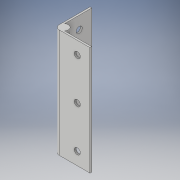
# Autodesk Inventor part: scharnier
Saved by Autodesk Inventor 2019 (Build 230136000, 136)
## iProperties
Created: 2018-06-15
Part Number: scharnier
Material: Generic
Document SubType Name: Modeling
Designer: daniel
Density: 1 g/cm^3
Appearance: Default
Author: daniel
Autodesk Inventor part; units mm, degrees
ref_plane "YZ Plane" through (0, 0, 0) normal (1, 0, 0) x (0, 1, 0)
ref_plane "XZ Plane" through (0, 0, 0) normal (0, 1, 0) x (-1, 0, 0)
ref_plane "XY Plane" through (0, 0, 0) normal (0, 0, 1) x (1, 0, 0)
sketch "Sketch1" plane through (0, 0, 0) normal (0, 1, 0) x (-1, 0, 0)
  circle A0 centre (0, 0) radius 2.5
  line L0 (-22.4, 0) -> (15.4, 0) projected
  line L1 (2.5, 0) -> (1.5, 0)
  line L2 (1.5, 0) -> (1.5, -17)
  line L3 (1.5, -17) -> (2.5, -17)
  line L4 (2.5, -17) -> (2.5, 0)
  line L5 (0, 0) -> (-7.0711, -7.0711) construction
  line L6 (0, 0) -> (10, 0) construction
  line L7 (0, 1.5) -> (-17, 1.5)
  line L8 (-17, 1.5) -> (-17, 2.5)
  line L9 (-17, 2.5) -> (0, 2.5)
  line L10 (0, 1.5) -> (0, 2.5)
  dimension "d0" = 5
  dimension "d1" = 1
  dimension "d2" = 17
  dimension "d3" = 10
  dimension "d4" = 135
  constraints: 20 end point, 4 symmetric about line, 2 horizontal, 2 parallel, 2 perpendicular, 1 coincident, 1 equal length, 1 horizontal alignment, 1 point on line, 2 other
  measures "d1" distance of L3.end L2.end
  measures "d2" distance of L2.end L1.end
  measures "d3" distance of L5.start L5.end
  measures "d4" angle of L5 L6
extrude "Extrusion1" add sketch "Sketch1" along normal blind 60
sketch "Sketch2" plane through (17, 0, 1.5) normal (0, 0, -1) x (-1, 0, 0)
  line L0 (0, 60) -> (15, 60) projected
  line L1 (7, 60) -> (7, 0) construction
  line L2 (15, 0) -> (0, 0) projected
  line L3 (0, 0) -> (0, 60) projected
  point P0 (17, 0)
  point P1 (7, 30)
  point P2 (7, 53)
  point P3 (7, 7)
  dimension "d7" = 7
  dimension "d8" = 30
  dimension "d9" = 7
  dimension "d10" = 7
  constraints: 4 point on line, 2 end point, 1 midpoint, 1 vertical
  measures "d7" distance between parallel lines of L3 L1
  measures "d8" distance from line of L0 point (7, 30)
  measures "d9" distance from line of L0 point (7, 53)
  measures "d10" distance from line of L2 point (7, 7)
hole "Hole1" at (10, 30, 1.5) at (10, 53, 1.5) at (10, 7, 1.5) direction (0, 0, 1) diameter 3.4 end through all clearance for "Countersunk Flat Head Screw DIN EN ISO 2009" size "M3" standard "DIN"
sketch "Sketch3" plane through (-1.5, 0, -2) normal (1, 0, 0) x (0, 0, -1)
  line L0 (0, 60) -> (15, 60) projected
  line L1 (8, 60) -> (8, 0) construction
  line L2 (15, 0) -> (15, 60) projected
  line L3 (15, 0) -> (0, 0) projected
  point P0 (-2, 0)
  point P1 (8, 30)
  point P2 (8, 7)
  point P3 (8, 53)
  dimension "d18" = 7
  dimension "d19" = 30
  dimension "d20" = 7
  dimension "d21" = 7
  constraints: 3 point on line, 2 end point, 1 midpoint, 1 vertical
  measures "d18" distance between parallel lines of L2 L1
  measures "d19" distance from line of L3 point (8, 30)
  measures "d20" distance from line of L3 point (8, 7)
  measures "d21" distance from line of L0 point (8, 53)
hole "Hole2" at (-1.5, 30, -10) at (-1.5, 7, -10) at (-1.5, 53, -10) direction (-1, 0, 0) diameter 3.4 end through all clearance for "Countersunk Flat Head Screw DIN EN ISO 2009" size "M3" standard "DIN"
body "Solid1"
